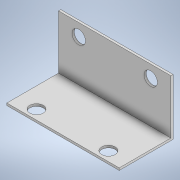
# Autodesk Inventor part: Hinge angle
Saved by Autodesk Inventor 2021 (Build 250183000, 183)
## iProperties
Created: 2023-05-31
Part Number: Hinge angle
Material: Generic
Document SubType Name: Modeling
Designer: shrus
Density: 1 g/cm^3
Appearance: Default
Author: shrus
Autodesk Inventor part; units mm, degrees
ref_plane "YZ Plane" through (0, 0, 0) normal (1, 0, 0) x (0, 1, 0)
ref_plane "XZ Plane" through (0, 0, 0) normal (0, 1, 0) x (-1, 0, 0)
ref_plane "XY Plane" through (0, 0, 0) normal (0, 0, 1) x (1, 0, 0)
sketch "Sketch1" plane through (0, 0, 0) normal (0, 0, 1) x (1, 0, 0)
  line L0 (-11.7965, 10.5077) -> (13.2035, 10.5077)
  line L1 (13.2035, 10.5077) -> (13.2035, -1.4923)
  line L2 (13.2035, -1.4923) -> (-11.7965, -1.4923)
  line L3 (-11.7965, -1.4923) -> (-11.7965, 10.5077)
  line L4 (-11.7965, -1.4923) -> (-11.7965, -1.9923)
  line L5 (-11.7965, -1.9923) -> (13.2035, -1.9923)
  circle A0 centre (-7.2965, 7.7152) radius 1.5
  circle A1 centre (8.7035, 7.7152) radius 1.5
  line L6 (13.2035, -1.4923) -> (13.2035, -1.9923)
  point P0 (0, 0)
  dimension "d0" = 25
  dimension "d1" = 12
  dimension "d7" = 3
  dimension "d8" = 3
  constraints: 14 end point, 4 perpendicular, 2 centre point, 1 horizontal, 1 parallel, 1 vertical
  measures "d0" distance of L0.start L0.end
  measures "d1" distance of L0.end L1.end
  measures "d7" diameter of A0
  measures "d8" diameter of A1
extrude "Extrusion1" add sketch "Sketch1" along normal blind 0.5 contours L0 L1 L2 L3
sketch "Sketch2" plane through (-11.7965, -1.4923, 0) normal (0, -1, 0) x (1, 0, 0)
  line L0 (25, 0) -> (0, 0) projected
  line L1 (0, 0) -> (0, 12)
  line L2 (0, 12) -> (25, 12)
  line L3 (25, 12) -> (25, 0)
  line L4 (25, 0) -> (0, 0)
  circle A0 centre (4.5, 9.9014) radius 1.5
  circle A1 centre (20.5, 9.9014) radius 1.5
  point P0 (11.7965, 0)
  dimension "d11" = 12
  dimension "d16" = 3
  dimension "d17" = 3
  constraints: 8 end point, 2 centre point, 2 perpendicular, 1 horizontal, 1 vertical
  measures "d11" distance of L0.end L1.end
  measures "d16" diameter of A0
  measures "d17" diameter of A1
extrude "Extrusion2" add sketch "Sketch2" along normal blind 0.5
body "Solid1"
